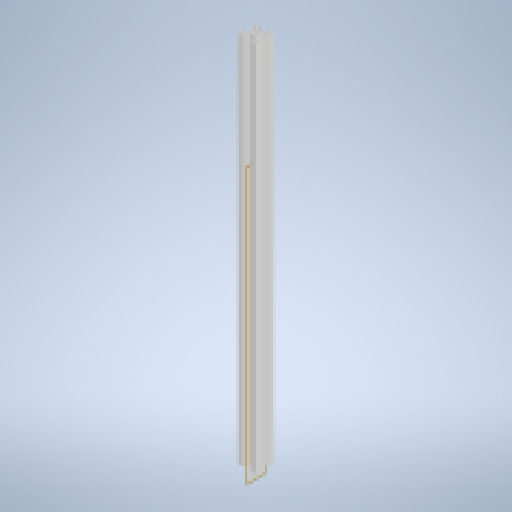
# Autodesk Inventor part: VSLOT 2040 Extrusion x 1m
Saved by Autodesk Inventor 2023 (Build 270158000, 158)
## iProperties
Created: 2020-07-22
Part Number: VSLOT 2040 Extrusion x 1m
Material: Aluminum 6061
Document SubType Name: Modeling
Designer: juanp
Density: 2.7 g/cm^3
Appearance: Aluminum - Dark
Mass: 278.306 g
Surface Area: 967.681 cm^2
Volume: 103.076 cm^3
Author: juanp
Autodesk Inventor part; units mm, degrees
ref_plane "YZ Plane" through (0, 0, 0) normal (1, 0, 0) x (0, 1, 0)
ref_plane "XZ Plane" through (0, 0, 0) normal (0, 1, 0) x (-1, 0, 0)
ref_plane "XY Plane" through (0, 0, 0) normal (0, 0, 1) x (1, 0, 0)
sketch "Sketch1" plane through (0, 0, 0) normal (0, 1, 0) x (-1, 0, 0)
  circle A0 centre (0, 0) radius 2.1
  line L0 (10, 10) -> (-10, 10) construction
  line L1 (-10, 10) -> (-10, -10) construction
  line L2 (-10, -10) -> (10, -10)
  line L3 (10, -10) -> (10, 10) construction
  line L4 (10, 10) -> (-10, -10) construction
  line L5 (-10, 10) -> (10, -10) construction
  line L6 (8.2, 10) -> (8.2, -10) construction
  line L7 (3.9, 10) -> (3.9, -10) construction
  line L8 (8.2, 3.125) -> (8.2, -3.125) construction
  line L9 (10, 4.58) -> (10, -4.58) construction
  line L10 (8.2, 5.5) -> (8.2, -5.5) construction
  line L11 (3.3697, 4.4303) -> (4.4303, 3.3697) construction
  line L12 (10, 10) -> (10, 4.58)
  line L13 (10, 4.58) -> (8.545, 3.125)
  line L14 (8.545, 3.125) -> (8.2, 3.125)
  line L15 (8.2, 3.125) -> (8.2, 5.5)
  line L16 (14, 0) -> (-14, 0) construction
  line L17 (8.2, 5.5) -> (6.5607, 5.5)
  line L18 (6.5607, 5.5) -> (3.9, 2.8393)
  line L19 (3.9, 2.8393) -> (3.9, 0)
  line L20 (10, -10) -> (10, -4.58)
  line L21 (10, -4.58) -> (8.545, -3.125)
  line L22 (8.545, -3.125) -> (8.2, -3.125)
  line L23 (8.2, -3.125) -> (8.2, -5.5)
  line L24 (8.2, -5.5) -> (6.5607, -5.5)
  line L25 (6.5607, -5.5) -> (3.9, -2.8393)
  line L26 (3.9, -2.8393) -> (3.9, 0)
  line L27 (-10, 10) -> (-4.58, 10)
  line L28 (-4.58, 10) -> (-3.125, 8.545)
  line L29 (-3.125, 8.2) -> (-5.5, 8.2)
  line L30 (-5.5, 8.2) -> (-5.5, 6.5607)
  line L31 (-5.5, 6.5607) -> (-2.8393, 3.9)
  line L32 (-2.8393, 3.9) -> (0, 3.9)
  line L33 (2.8393, 3.9) -> (0, 3.9)
  line L34 (5.5, 6.5607) -> (2.8393, 3.9)
  line L35 (5.5, 8.2) -> (5.5, 6.5607)
  line L36 (3.125, 8.2) -> (5.5, 8.2)
  line L37 (3.125, 8.545) -> (3.125, 8.2)
  line L38 (4.58, 10) -> (3.125, 8.545)
  line L39 (-3.125, 8.545) -> (-3.125, 8.2)
  line L40 (10, 10) -> (4.58, 10)
  line L41 (-10, -10) -> (-10, -4.58)
  line L42 (-10, -4.58) -> (-8.545, -3.125)
  line L43 (-8.2, -3.125) -> (-8.2, -5.5)
  line L44 (-8.2, -5.5) -> (-6.5607, -5.5)
  line L45 (-6.5607, -5.5) -> (-3.9, -2.8393)
  line L46 (-3.9, -2.8393) -> (-3.9, 0)
  line L47 (-3.9, 2.8393) -> (-3.9, 0)
  line L48 (-6.5607, 5.5) -> (-3.9, 2.8393)
  line L49 (-8.2, 5.5) -> (-6.5607, 5.5)
  line L50 (-8.2, 3.125) -> (-8.2, 5.5)
  line L51 (-8.545, 3.125) -> (-8.2, 3.125)
  line L52 (-10, 4.58) -> (-8.545, 3.125)
  line L53 (-8.545, -3.125) -> (-8.2, -3.125)
  line L54 (-10, 10) -> (-10, 4.58)
  line L55 (10, -10) -> (4.58, -10) construction
  line L56 (4.58, -10) -> (3.125, -8.545)
  line L57 (3.125, -8.2) -> (5.5, -8.2)
  line L58 (5.5, -8.2) -> (5.5, -6.5607)
  line L59 (5.5, -6.5607) -> (2.8393, -3.9)
  line L60 (2.8393, -3.9) -> (0, -3.9)
  line L61 (-2.8393, -3.9) -> (0, -3.9)
  line L62 (-5.5, -6.5607) -> (-2.8393, -3.9)
  line L63 (-5.5, -8.2) -> (-5.5, -6.5607)
  line L64 (-3.125, -8.2) -> (-5.5, -8.2)
  line L65 (-3.125, -8.545) -> (-3.125, -8.2)
  line L66 (-4.58, -10) -> (-3.125, -8.545)
  line L67 (3.125, -8.545) -> (3.125, -8.2)
  line L68 (-10, -10) -> (-4.58, -10) construction
  line L69 (5.5, -6.5607) -> (6.2393, -7.3)
  line L70 (6.2393, -7.3) -> (8.2, -7.3)
  line L71 (0, -10) -> (0, -9) construction
  line L72 (-5.5, -6.5607) -> (-6.2393, -7.3)
  line L73 (-6.2393, -7.3) -> (-8.2, -7.3)
  line L74 (8.2, -7.3) -> (8.2, -10)
  line L75 (-8.2, -7.3) -> (-8.2, -10)
  circle A1 centre (0, -20) radius 2.1
  line L76 (10, -30) -> (10, -24.58)
  line L77 (10, -24.58) -> (8.545, -23.125)
  line L78 (8.545, -23.125) -> (8.2, -23.125)
  line L79 (8.2, -23.125) -> (8.2, -25.5)
  line L80 (8.2, -25.5) -> (6.5607, -25.5)
  line L81 (6.5607, -25.5) -> (3.9, -22.8393)
  line L82 (3.9, -22.8393) -> (3.9, -20)
  line L83 (10, -10) -> (10, -15.42)
  line L84 (10, -15.42) -> (8.545, -16.875)
  line L85 (8.2, -16.875) -> (8.2, -14.5)
  line L86 (8.2, -14.5) -> (6.5607, -14.5)
  line L87 (6.5607, -14.5) -> (3.9, -17.1607)
  line L88 (3.9, -17.1607) -> (3.9, -20)
  line L89 (-10, -30) -> (-4.58, -30)
  line L90 (-4.58, -30) -> (-3.125, -28.545)
  line L91 (-3.125, -28.2) -> (-5.5, -28.2)
  line L92 (-5.5, -28.2) -> (-5.5, -26.5607)
  line L93 (-5.5, -26.5607) -> (-2.8393, -23.9)
  line L94 (-2.8393, -23.9) -> (0, -23.9)
  line L95 (2.8393, -23.9) -> (0, -23.9)
  line L96 (5.5, -26.5607) -> (2.8393, -23.9)
  line L97 (5.5, -28.2) -> (5.5, -26.5607)
  line L98 (3.125, -28.2) -> (5.5, -28.2)
  line L99 (3.125, -28.545) -> (3.125, -28.2)
  line L100 (4.58, -30) -> (3.125, -28.545)
  line L101 (-3.125, -28.545) -> (-3.125, -28.2)
  line L102 (10, -30) -> (4.58, -30)
  line L103 (-10, -10) -> (-10, -15.42)
  line L104 (-10, -15.42) -> (-8.545, -16.875)
  line L105 (-8.2, -16.875) -> (-8.2, -14.5)
  line L106 (-8.2, -14.5) -> (-6.5607, -14.5)
  line L107 (-6.5607, -14.5) -> (-3.9, -17.1607)
  line L108 (-3.9, -17.1607) -> (-3.9, -20)
  line L109 (-3.9, -22.8393) -> (-3.9, -20)
  line L110 (-6.5607, -25.5) -> (-3.9, -22.8393)
  line L111 (-8.2, -25.5) -> (-6.5607, -25.5)
  line L112 (-8.2, -23.125) -> (-8.2, -25.5)
  line L113 (-8.545, -23.125) -> (-8.2, -23.125)
  line L114 (-10, -24.58) -> (-8.545, -23.125)
  line L115 (-8.545, -16.875) -> (-8.2, -16.875)
  line L116 (-10, -30) -> (-10, -24.58)
  line L117 (5.5, -13.4393) -> (2.8393, -16.1)
  line L118 (2.8393, -16.1) -> (0, -16.1)
  line L119 (-2.8393, -16.1) -> (0, -16.1)
  line L120 (-5.5, -13.4393) -> (-2.8393, -16.1)
  line L121 (5.5, -13.4393) -> (6.2393, -12.7)
  line L122 (6.2393, -12.7) -> (8.2, -12.7)
  line L123 (-5.5, -13.4393) -> (-6.2393, -12.7)
  line L124 (-6.2393, -12.7) -> (-8.2, -12.7)
  line L125 (8.2, -12.7) -> (8.2, -10)
  line L126 (-8.2, -12.7) -> (-8.2, -10)
  line L127 (8.545, -16.875) -> (8.2, -16.875)
  point P0 (10, 0)
  point P1 (8.2, 0)
  point P2 (3.9, 3.9)
  point P3 (-3.3697, 4.4303)
  point P4 (-4.4303, -3.3697)
  point P5 (3.3697, -4.4303)
  dimension "d0" = 4.2
  dimension "d1" = 20
  dimension "d2" = 20
  dimension "d3" = 1.8
  dimension "d4" = 4.3
  dimension "d5" = 6.25
  dimension "d6" = 9.16
  dimension "d7" = 11
  dimension "d8" = 1.5
  dimension "d9" = 45
  dimension "d12" = 360
  dimension "d17" = 1.8
  dimension "d18" = 1
  constraints: 254 end point, 58 symmetric about line, 15 point on line, 10 midpoint, 8 perpendicular, 5 vertical, 3 horizontal, 2 centre point, 2 collinear, 2 parallel, 1 coincident, 122 other
  measures "d0" diameter of A0
  measures "d1" distance of L2.end L1.end
  measures "d2" distance of L1.end L0.end
  measures "d3" distance between parallel lines of L6 L3
  measures "d4" distance between parallel lines of L7 L6
  measures "d5" distance of L8.start L8.end
  measures "d6" distance of L9.start L9.end
  measures "d7" distance of L10.start L10.end
  measures "d8" distance of L11.start L11.end
  measures "d9" angle of L16 L13
  measures "d17" distance between parallel lines of L24 L70
  measures "d18" distance of L71.start L71.end
extrude "Extrusion1" add sketch "Sketch1" along normal blind 425 contours L41 L42 L53 L43 L44 L45 L46 L47 L48 L49 L50 L51 L52 L54 L27 L28 L39 L29 L30 L31 L32 L33 L34 L35 L36 L37 L38 L40 L12 L13 L14 L15 L17 L18 L19 L26 L25 L24 L23 L22 L21 L20 L2 L74 L70 L69 L59 L60 L61 L62 L72 L73 L75 | L75 L73 L72 L63 L64 L65 L66 L2 | L56 L67 L57 L58 L69 L70 L74 L2
ref_plane "Work Plane1" through (-2.8393, 0, 0) normal (0, 0, -1) x (-1, 0, 0)
ref_plane "Work Plane2" through (0, 0, 4.58) normal (1, 0, 0) x (0, 0, -1)
ref_plane "Work Plane3" through (0, 212.5, 0) normal (0, 1, 0) x (1, 0, 0)
ref_plane "Work Plane5" through (0, 212.5, 0) normal (0, -1, 0) x (1, 0, 0)
ref_plane "Work Plane7" through (0, 0, 4.58) normal (1, 0, 0) x (0, 0, -1)
ref_plane "Plano de trabajo8" through (0, 0, -10) normal (1, 0, 0) x (0, 0, -1)
body "Solid1"
